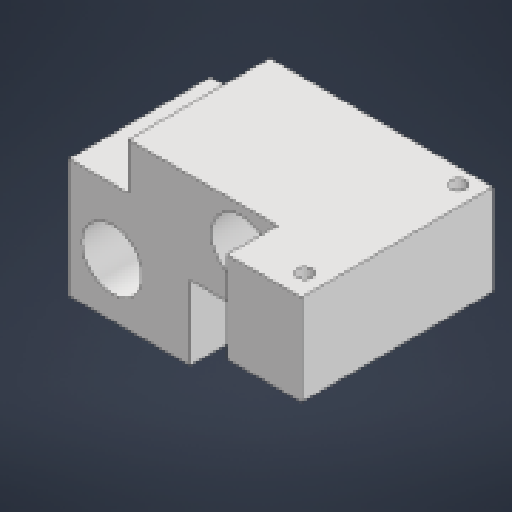
# Autodesk Inventor part: 固定传动
Saved by Autodesk Inventor 2025 (Build 290162000, 162)
## iProperties
Created: 2025-12-09
Part Number: 固定传动
Material: 常规
Document SubType Name: Modeling
Designer: XH
Density: 1 g/cm^3
Appearance: 默认
Author: XH
Autodesk Inventor part; units mm, degrees
ref_plane "YZ Plane" through (0, 0, 0) normal (1, 0, 0) x (0, 1, 0)
ref_plane "XZ Plane" through (0, 0, 0) normal (0, 1, 0) x (-1, 0, 0)
ref_plane "XY Plane" through (0, 0, 0) normal (0, 0, 1) x (1, 0, 0)
sketch "草图1" plane through (0, 0, 0) normal (0, 0, 1) x (1, 0, 0)
  line L0 (-22.2679, -12.5636) -> (3.7321, -12.5636) projected
  line L1 (-24.2679, 7.4364) -> (5.7321, 7.4364)
  line L2 (5.7321, 7.4364) -> (5.7321, -12.5636)
  line L3 (5.7321, -12.5636) -> (-24.2679, -12.5636)
  line L4 (-24.2679, -12.5636) -> (-24.2679, 7.4364)
  point P0 (-22.2679, -12.5636)
  point P1 (3.7321, -12.5636)
  dimension "d4" = 30
  dimension "d5" = 20
  constraints: 8 end point, 2 parallel, 1 collinear, 1 horizontal, 1 perpendicular
  measures "d4" distance of L1.start L1.end
  measures "d5" distance of L1.end L2.end
extrude "拉伸1" add sketch "草图1" along normal blind 19
sketch "草图2" plane through (0, 0, 0) normal (0, 0, -1) x (-1, 0, 0)
  line L0 (24.2679, 7.4364) -> (24.2679, -12.5636) projected
  line L1 (24.2679, -12.5636) -> (31.2679, -12.5636)
  line L2 (31.2679, -12.5636) -> (31.2679, -0.5636)
  line L3 (31.2679, -0.5636) -> (24.2679, -0.5636)
  line L4 (24.2679, -0.5636) -> (24.2679, -12.5636)
  point P0 (0, 0)
  dimension "d6" = 7
  dimension "d7" = 12
  constraints: 8 end point, 2 parallel, 1 horizontal, 1 perpendicular
  measures "d6" distance of L2.end L3.end
  measures "d7" distance of L1.end L2.end
extrude "拉伸2" add sketch "草图2" against normal up to surface (19 mm away)
sketch "草图3" plane through (0, 0, 0) normal (0, 0, -1) x (-1, 0, 0)
  circle A0 centre (-0.6256, 1.5535) radius 3
  circle A1 centre (26.4728, -5.3671) radius 4.025
  point P0 (0, 0)
  dimension "d10" = 6
  dimension "d11" = 8.05
  constraints: 2 centre point
  measures "d10" diameter of A0
  measures "d11" diameter of A1
extrude "拉伸3" cut sketch "草图3" against normal blind 40
sketch "草图4" plane through (5.7321, -12.5636, 0) normal (1, 0, 0) x (0, 0, -1)
  line L0 (-19, 0) -> (-4, 0)
  line L1 (-4, 0) -> (-4, 10)
  line L2 (-4, 10) -> (-19, 10)
  line L3 (-19, 10) -> (-19, 0)
  point P0 (0, 12.5636)
  dimension "d14" = 10
  dimension "d15" = 15
  constraints: 8 end point, 2 parallel, 1 horizontal, 1 perpendicular
  measures "d14" distance of L2.end L0.start
  measures "d15" distance of L1.end L2.end
extrude "拉伸4" cut sketch "草图4" against normal blind 21.75
chamfer "倒角1" distance 4 angle 45 1 edges at (-24.2679, -0.5636, 9.5)
sketch "草图5" plane through (5.7321, -12.5636, 0) normal (1, 0, 0) x (0, 0, -1)
  line L0 (-4, 0) -> (-19, 0) projected
  line L1 (-4, 0) -> (0, 0)
  line L2 (0, 0) -> (0, 10)
  line L3 (0, 10) -> (-4, 10)
  line L4 (-4, 10) -> (-4, 0)
  line L5 (0, 0) -> (0, 20) projected
  line L6 (-19, 10) -> (-4, 10) projected
  point P0 (0, 12.5636)
  constraints: 8 end point, 2 collinear, 2 parallel, 1 horizontal, 1 perpendicular
extrude "拉伸5" cut sketch "草图5" against normal blind 10
sketch "草图6" plane through (5.7321, -2.5636, 0) normal (0, -1, 0) x (1, 0, 0)
  line L0 (0, 0) -> (0, 19) projected
  line L1 (0, 0) -> (-8, 0)
  line L2 (-8, 0) -> (-8, 25.7509)
  line L3 (-8, 25.7509) -> (0, 25.7509)
  line L4 (0, 25.7509) -> (0, 0)
  line L5 (-12.3, 25.7509) -> (0, 25.7509) projected
  line L6 (-21.75, 19) -> (0, 19) projected
  line L7 (-8, 25.7509) -> (-10, 25.7509)
  line L8 (-10, 25.7509) -> (-10, 19)
  line L9 (-10, 19) -> (-8, 19)
  line L10 (-8, 19) -> (-8, 25.7509)
  point P0 (-5.7321, 0)
  point P1 (-8, 19)
  dimension "d23" = 8
  dimension "d28" = 10
  constraints: 16 end point, 4 parallel, 2 horizontal, 2 perpendicular, 1 collinear, 1 point on line
  measures "d23" distance between parallel lines of L2 L4
  measures "d28" distance between parallel lines of L4 L8
extrude "拉伸6" add sketch "草图6" against normal up to surface (10 mm away)
sketch "草图8" plane through (0, 0, 0) normal (0, 0, -1) x (-1, 0, 0)
  circle A0 centre (-0.6256, 1.5535) radius 3
  point P0 (0, 0)
  constraints: 1 centre point, 2 other
extrude "拉伸7" cut sketch "草图8" against normal blind 42.75
fillet "圆角1" radius 4 1 edges at (-4.2679, 2.4364, 19)
sketch "草图9" plane through (0, 0, 0) normal (0, 0, -1) x (-1, 0, 0)
  circle A0 centre (9.0791, 4.3462) radius 4.025
  point P0 (0, 0)
  dimension "d35" = 8.05
  constraints: 1 centre point, 1 other
  measures "d35" diameter of A0
extrude "拉伸8" cut sketch "草图9" against normal blind 33.75
delete faces "删除1" heal yes whole lump no faces at (-4.5427, 0.7697, 21.5431)
delete faces "删除2" heal yes whole lump no faces at (-1.434, 3.7348, 17.1673)
offset faces "大小1" outward 3 faces at (2.3988, 7.4364, 14.917) (-15.8614, 7.4364, 6.3333)
sketch "草图10" plane through (-16.0179, -2.5636, 19) normal (0, -1, 0) x (1, 0, 0)
  ellipse E0 centre (19.1097, 3.7017) end of major axis (18.1097, 3.7017) minor radius 1 projected
  ellipse E1 centre (19.1586, -16.9435) end of major axis (18.1586, -16.9435) minor radius 1 projected
  point P0 (16.0179, -19)
  constraints: 2 other
extrude "拉伸9" cut sketch "草图10" against normal blind 33.75
offset faces "大小2" outward 1 faces at (-31.2679, -8.5636, 6.3333)
offset faces "大小3" outward 4 faces at (-30.9346, -0.5636, 6.3333)
sketch "草图11" plane through (-4.2679, -2.5636, 25.7509) normal (0, 0, 1) x (1, 0, 0)
  line L0 (10, 13) -> (-20, 13) projected
  line L1 (10, 13) -> (-20.4657, 13)
  line L2 (-20.4657, 13) -> (-20.4657, 12.2117)
  line L3 (-20.4657, 12.2117) -> (10, 12.2117)
  line L4 (10, 12.2117) -> (10, 13)
  line L5 (-8.462, 12.203) -> (17.6165, 12.2153)
  point P0 (4.2679, 2.5636)
  constraints: 10 end point, 2 parallel, 1 horizontal, 1 perpendicular, 1 point on line, 3 other
extrude "拉伸10" cut sketch "草图11" against normal blind 36.75
